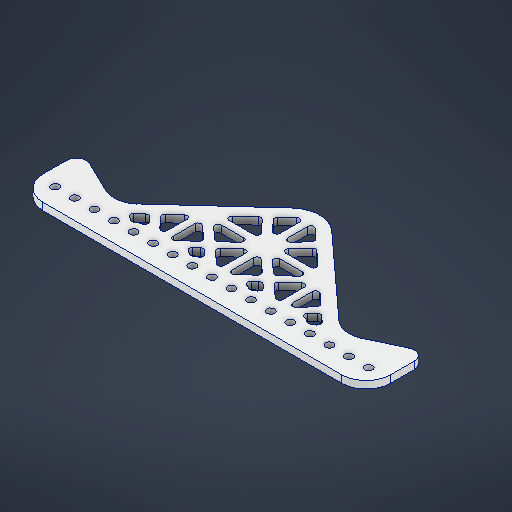
# Autodesk Inventor part: cage-brace
Saved by Autodesk Inventor 2025.1 (Build 291241020, 241B)
## iProperties
Created: 2025-03-18
Part Number: cage-brace
Material: Aluminum 6061
Document SubType Name: Sheet Metal
Designer: mathe
Density: 2.7 g/cm^3
Sheet Metal Rule: Default
Appearance: Aluminum - Flat
Author: mathe
Autodesk Inventor part; units mm, degrees
ref_plane "YZ Plane" through (0, 0, 0) normal (1, 0, 0) x (0, 1, 0)
ref_plane "XZ Plane" through (0, 0, 0) normal (0, 1, 0) x (-1, 0, 0)
ref_plane "XY Plane" through (0, 0, 0) normal (0, 0, 1) x (1, 0, 0)
sketch "Sketch2" plane through (0, 0, 0) normal (0, 1, 0) x (-1, 0, 0)
  line L0 (193.675, 0) -> (0, 0)
  arc A0 (0, 0) -> (-15.875, -15.875) centre (0, -15.875) ccw
  line L1 (-15.875, -15.875) -> (-15.875, -31.1578)
  arc A1 (-15.875, -31.1578) -> (-6.7641, -36.8762) centre (-9.525, -31.1578) ccw
  line L2 (-6.7641, -36.8762) -> (13.7353, -26.979)
  arc A2 (31.3347, -29.5453) -> (13.7353, -26.979) centre (20.6375, -41.275) ccw
  line L3 (31.3347, -29.5453) -> (84.0009, -77.5756)
  arc A3 (84.0009, -77.5756) -> (109.6741, -77.5756) centre (96.8375, -63.5) ccw
  line L4 (109.6741, -77.5756) -> (162.3403, -29.5453)
  arc A4 (179.9397, -26.979) -> (162.3403, -29.5453) centre (173.0375, -41.275) ccw
  line L5 (179.9397, -26.979) -> (200.4391, -36.8762)
  arc A5 (200.4391, -36.8762) -> (209.55, -31.1578) centre (203.2, -31.1578) ccw
  line L6 (209.55, -31.1578) -> (209.55, -15.875)
  arc A6 (209.55, -15.875) -> (193.675, 0) centre (193.675, -15.875) ccw
  arc A7 (137.4775, -37.2895) -> (140.84, -38.7687) centre (139.4841, -37.2895) ccw
  line L7 (137.4775, -37.2895) -> (137.4775, -24.3884)
  arc A8 (140.9633, -23.0325) -> (137.4775, -24.3884) centre (139.4841, -24.3884) ccw
  line L8 (140.9633, -23.0325) -> (147.3895, -30.0429)
  arc A9 (147.2662, -32.878) -> (147.3895, -30.0429) centre (145.9103, -31.3988) ccw
  line L9 (147.2662, -32.878) -> (140.84, -38.7687)
  arc A10 (117.2434, -34.8511) -> (114.5316, -34.8511) centre (115.8875, -36.3303) ccw
  line L10 (117.2434, -34.8511) -> (124.605, -41.5992)
  arc A11 (123.2491, -45.085) -> (124.605, -41.5992) centre (123.2491, -43.0784) ccw
  line L11 (123.2491, -45.085) -> (108.5259, -45.085)
  arc A12 (107.17, -41.5992) -> (108.5259, -45.085) centre (108.5259, -43.0784) ccw
  line L12 (107.17, -41.5992) -> (114.5316, -34.8511)
  arc A13 (64.64, -21.5563) -> (61.2775, -23.0355) centre (63.2841, -23.0355) ccw
  line L13 (64.64, -21.5563) -> (72.4149, -28.6833)
  arc A14 (72.4149, -31.6417) -> (72.4149, -28.6833) centre (71.059, -30.1625) ccw
  line L14 (72.4149, -31.6417) -> (64.64, -38.7687)
  arc A15 (61.2775, -37.2895) -> (64.64, -38.7687) centre (63.2841, -37.2895) ccw
  line L15 (61.2775, -37.2895) -> (61.2775, -23.0355)
  arc A16 (99.3775, -37.2895) -> (102.74, -38.7687) centre (101.3841, -37.2895) ccw
  line L16 (99.3775, -37.2895) -> (99.3775, -23.0355)
  arc A17 (102.74, -21.5563) -> (99.3775, -23.0355) centre (101.3841, -23.0355) ccw
  line L17 (102.74, -21.5563) -> (110.5149, -28.6833)
  arc A18 (110.5149, -31.6417) -> (110.5149, -28.6833) centre (109.159, -30.1625) ccw
  line L18 (110.5149, -31.6417) -> (102.74, -38.7687)
  arc A19 (112.4883, -19.7393) -> (111.9081, -23.069) centre (113.264, -21.5898) ccw
  arc A20 (112.4883, -19.7393) -> (114.5656, -18.4425) centre (109.5375, -12.7) ccw
  arc A21 (117.2094, -18.4425) -> (114.5656, -18.4425) centre (115.8875, -19.9521) ccw
  arc A22 (117.2094, -18.4425) -> (119.2867, -19.7393) centre (122.2375, -12.7) ccw
  arc A23 (119.8669, -23.069) -> (119.2867, -19.7393) centre (118.511, -21.5898) ccw
  line L19 (119.8669, -23.069) -> (117.2434, -25.4739)
  arc A24 (114.5316, -25.4739) -> (117.2434, -25.4739) centre (115.8875, -23.9947) ccw
  line L20 (114.5316, -25.4739) -> (111.9081, -23.069)
  line L21 (107.173, -50.165) -> (123.2491, -50.165)
  arc A25 (124.605, -53.6508) -> (123.2491, -50.165) centre (123.2491, -52.1716) ccw
  line L22 (124.605, -53.6508) -> (115.8693, -61.6585)
  arc A26 (113.0342, -61.5352) -> (115.8693, -61.6585) centre (114.5134, -60.1793) ccw
  line L23 (113.0342, -61.5352) -> (105.6938, -53.5275)
  arc A27 (107.173, -50.165) -> (105.6938, -53.5275) centre (107.173, -52.1716) ccw
  line L24 (109.1662, -67.803) -> (102.74, -73.6937)
  arc A28 (99.3775, -72.2145) -> (102.74, -73.6937) centre (101.3841, -72.2145) ccw
  line L25 (99.3775, -72.2145) -> (99.3775, -59.3134)
  arc A29 (102.8633, -57.9575) -> (99.3775, -59.3134) centre (101.3841, -59.3134) ccw
  line L26 (102.8633, -57.9575) -> (109.2895, -64.9679)
  arc A30 (109.1662, -67.803) -> (109.2895, -64.9679) centre (107.8103, -66.3238) ccw
  line L27 (70.4259, -50.165) -> (86.502, -50.165)
  arc A31 (87.9812, -53.5275) -> (86.502, -50.165) centre (86.502, -52.1716) ccw
  line L28 (87.9812, -53.5275) -> (80.6408, -61.5352)
  arc A32 (77.8057, -61.6585) -> (80.6408, -61.5352) centre (79.1616, -60.1793) ccw
  line L29 (77.8057, -61.6585) -> (69.07, -53.6508)
  arc A33 (70.4259, -50.165) -> (69.07, -53.6508) centre (70.4259, -52.1716) ccw
  line L30 (90.935, -73.6937) -> (84.5088, -67.803)
  arc A34 (84.3855, -64.9679) -> (84.5088, -67.803) centre (85.8647, -66.3238) ccw
  line L31 (84.3855, -64.9679) -> (90.8117, -57.9575)
  arc A35 (94.2975, -59.3134) -> (90.8117, -57.9575) centre (92.2909, -59.3134) ccw
  line L32 (94.2975, -59.3134) -> (94.2975, -72.2145)
  arc A36 (90.935, -73.6937) -> (94.2975, -72.2145) centre (92.2909, -72.2145) ccw
  line L33 (94.2975, -23.0355) -> (94.2975, -37.2895)
  arc A37 (90.935, -38.7687) -> (94.2975, -37.2895) centre (92.2909, -37.2895) ccw
  line L34 (90.935, -38.7687) -> (83.1601, -31.6417)
  arc A38 (83.1601, -28.6833) -> (83.1601, -31.6417) centre (84.516, -30.1625) ccw
  line L35 (83.1601, -28.6833) -> (90.935, -21.5563)
  arc A39 (94.2975, -23.0355) -> (90.935, -21.5563) centre (92.2909, -23.0355) ccw
  arc A40 (74.3883, -19.7393) -> (73.8081, -23.069) centre (75.164, -21.5898) ccw
  arc A41 (74.3883, -19.7393) -> (76.4656, -18.4425) centre (71.4375, -12.7) ccw
  arc A42 (79.1094, -18.4425) -> (76.4656, -18.4425) centre (77.7875, -19.9521) ccw
  arc A43 (79.1094, -18.4425) -> (81.1867, -19.7393) centre (84.1375, -12.7) ccw
  arc A44 (81.7669, -23.069) -> (81.1867, -19.7393) centre (80.411, -21.5898) ccw
  line L36 (81.7669, -23.069) -> (79.1434, -25.4739)
  arc A45 (76.4316, -25.4739) -> (79.1434, -25.4739) centre (77.7875, -23.9947) ccw
  line L37 (76.4316, -25.4739) -> (73.8081, -23.069)
  line L38 (46.2855, -30.0429) -> (52.7117, -23.0325)
  arc A46 (56.1975, -24.3884) -> (52.7117, -23.0325) centre (54.1909, -24.3884) ccw
  line L39 (56.1975, -24.3884) -> (56.1975, -37.2895)
  arc A47 (52.835, -38.7687) -> (56.1975, -37.2895) centre (54.1909, -37.2895) ccw
  line L40 (52.835, -38.7687) -> (46.4088, -32.878)
  arc A48 (46.2855, -30.0429) -> (46.4088, -32.878) centre (47.7647, -31.3988) ccw
  line L41 (79.1434, -34.8511) -> (86.505, -41.5992)
  arc A49 (85.1491, -45.085) -> (86.505, -41.5992) centre (85.1491, -43.0784) ccw
  line L42 (85.1491, -45.085) -> (70.4259, -45.085)
  arc A50 (69.07, -41.5992) -> (70.4259, -45.085) centre (70.4259, -43.0784) ccw
  line L43 (69.07, -41.5992) -> (76.4316, -34.8511)
  arc A51 (79.1434, -34.8511) -> (76.4316, -34.8511) centre (77.7875, -36.3303) ccw
  arc A52 (36.2883, -19.7393) -> (35.7081, -23.069) centre (37.064, -21.5898) ccw
  arc A53 (36.2883, -19.7393) -> (38.3656, -18.4425) centre (33.3375, -12.7) ccw
  arc A54 (41.0094, -18.4425) -> (38.3656, -18.4425) centre (39.6875, -19.9521) ccw
  arc A55 (41.0094, -18.4425) -> (44.3802, -20.1506) centre (46.0375, -12.7) ccw
  arc A56 (45.4237, -23.4652) -> (44.3802, -20.1506) centre (43.9445, -22.1093) ccw
  line L44 (45.4237, -23.4652) -> (42.5408, -26.6102)
  arc A57 (39.7057, -26.7335) -> (42.5408, -26.6102) centre (41.0616, -25.2543) ccw
  line L45 (39.7057, -26.7335) -> (35.7081, -23.069)
  line L46 (129.035, -38.7687) -> (121.2601, -31.6417)
  arc A58 (121.2601, -28.6833) -> (121.2601, -31.6417) centre (122.616, -30.1625) ccw
  line L47 (121.2601, -28.6833) -> (129.035, -21.5563)
  arc A59 (132.3975, -23.0355) -> (129.035, -21.5563) centre (130.3909, -23.0355) ccw
  line L48 (132.3975, -23.0355) -> (132.3975, -37.2895)
  arc A60 (129.035, -38.7687) -> (132.3975, -37.2895) centre (130.3909, -37.2895) ccw
  arc A61 (149.2948, -20.1506) -> (148.2513, -23.4652) centre (149.7305, -22.1093) ccw
  arc A62 (149.2948, -20.1506) -> (152.6656, -18.4425) centre (147.6375, -12.7) ccw
  arc A63 (155.3094, -18.4425) -> (152.6656, -18.4425) centre (153.9875, -19.9521) ccw
  arc A64 (155.3094, -18.4425) -> (157.3867, -19.7393) centre (160.3375, -12.7) ccw
  arc A65 (157.9669, -23.069) -> (157.3867, -19.7393) centre (156.611, -21.5898) ccw
  line L49 (157.9669, -23.069) -> (153.9693, -26.7335)
  arc A66 (151.1342, -26.6102) -> (153.9693, -26.7335) centre (152.6134, -25.2543) ccw
  line L50 (151.1342, -26.6102) -> (148.2513, -23.4652)
  circle A67 centre (185.7375, -12.7) radius 2.5527
  circle A68 centre (198.4375, -12.7) radius 2.5527
  circle A69 centre (-4.7625, -12.7) radius 2.5527
  circle A70 centre (134.9375, -12.7) radius 2.5527
  circle A71 centre (122.2375, -12.7) radius 2.5527
  circle A72 centre (109.5375, -12.7) radius 2.5527
  circle A73 centre (96.8375, -12.7) radius 2.5527
  circle A74 centre (84.1375, -12.7) radius 2.5527
  circle A75 centre (71.4375, -12.7) radius 2.5527
  circle A76 centre (58.7375, -12.7) radius 2.5527
  circle A77 centre (46.0375, -12.7) radius 2.5527
  circle A78 centre (33.3375, -12.7) radius 2.5527
  circle A79 centre (20.6375, -12.7) radius 2.5527
  circle A80 centre (160.3375, -12.7) radius 2.5527
  circle A81 centre (173.0375, -12.7) radius 2.5527
  circle A82 centre (147.6375, -12.7) radius 2.5527
  circle A83 centre (7.9375, -12.7) radius 2.5527
  point P0 (179.9397, -26.979)
  point P1 (-15.875, -15.875)
  point P2 (-6.7641, -36.8762)
  point P3 (13.7353, -26.979)
  point P4 (155.3094, -18.4425)
  point P5 (157.3867, -19.7393)
  point P6 (157.9669, -23.069)
  point P7 (151.1342, -26.6102)
  point P8 (152.6656, -18.4425)
  point P9 (132.3975, -23.0355)
  point P10 (121.2601, -28.6833)
  point P11 (41.0094, -18.4425)
  point P12 (44.3802, -20.1506)
  point P13 (35.7081, -23.069)
  point P14 (38.3656, -18.4425)
  point P15 (79.1094, -18.4425)
  point P16 (81.7669, -23.069)
  point P17 (76.4316, -25.4739)
  point P18 (73.8081, -23.069)
  point P19 (76.4656, -18.4425)
  point P20 (87.9812, -53.5275)
  point P21 (102.8633, -57.9575)
  point P22 (124.605, -53.6508)
  point P23 (117.2094, -18.4425)
  point P24 (119.2867, -19.7393)
  point P25 (119.8669, -23.069)
  point P26 (114.5316, -25.4739)
  point P27 (111.9081, -23.069)
  point P28 (112.4883, -19.7393)
  point P29 (114.5656, -18.4425)
  point P30 (102.74, -21.5563)
  point P31 (110.5149, -31.6417)
  point P32 (102.74, -38.7687)
  point P33 (99.3775, -37.2895)
  point P34 (72.4149, -31.6417)
  point P35 (61.2775, -23.0355)
  point P36 (64.64, -21.5563)
  point P37 (123.2491, -45.085)
  point P38 (107.17, -41.5992)
  point P39 (114.5316, -34.8511)
  point P40 (117.2434, -34.8511)
  point P41 (140.9633, -23.0325)
  point P42 (147.2662, -32.878)
  point P43 (140.84, -38.7687)
extrude "Plate2" add sketch "Sketch2" along normal blind 4.7625
equation "\"d13\" = Thickness"
equation "\"BendRadius\" = Thickness"
equation "\"BendReliefWidth\" = Thickness"
equation "\"BendReliefDepth\" = 0.5 * Thickness"
equation "\"CornerReliefSize\" = 4 * Thickness"
equation "\"MinimumRemnant\" = 2 * Thickness"
equation "\"TransitionRadius\" = BendRadius"
equation "\"JacobiRadiusSize\" = BendRadius"
equation "\"GapSize\" = Thickness"
equation "\"Thickness\" = 4.7625"
body "Solid2"
